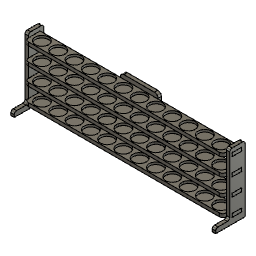
BDPRackv2 (Autodesk Fusion 360 design; units mm, degrees)
Autodesk Fusion 360 part; units mm, degrees
sketch "Sketch1" plane through (0, 0, 0) normal (0, 1, 0) x (1, 0, 0)
  line L0 (0, 0) -> (1066.8, 0)
  line L1 (1066.8, 0) -> (1066.8, -82.55)
  line L2 (1066.8, -82.55) -> (0, -82.55)
  line L3 (0, -82.55) -> (0, 0)
  line L4 (0, 0) -> (-18.288, 0)
  line L5 (-18.288, 0) -> (-18.288, -50.8)
  line L6 (-18.288, -50.8) -> (0, -50.8)
  line L7 (0, -50.8) -> (0, 0)
  line L8 (1066.8, 0) -> (1085.088, 0)
  line L9 (1085.088, 0) -> (1085.088, -50.8)
  line L10 (1085.088, -50.8) -> (1066.8, -50.8)
  line L11 (1066.8, -50.8) -> (1066.8, 0)
  line L12 (0, 0) -> (50.8, 0) construction
  line L13 (50.8, 0) -> (50.8, -41.275) construction
  circle A0 centre (50.8, -41.275) radius 36.195
  circle A1 centre (138.5455, -41.275) radius 36.195
  circle A2 centre (226.2909, -41.275) radius 36.195
  circle A3 centre (314.0364, -41.275) radius 36.195
  circle A4 centre (401.7818, -41.275) radius 36.195
  circle A5 centre (489.5273, -41.275) radius 36.195
  circle A6 centre (577.2727, -41.275) radius 36.195
  circle A7 centre (665.0182, -41.275) radius 36.195
  circle A8 centre (752.7636, -41.275) radius 36.195
  circle A9 centre (840.5091, -41.275) radius 36.195
  circle A10 centre (928.2545, -41.275) radius 36.195
  circle A11 centre (1016, -41.275) radius 36.195
  dimension "d1" = 1066.8
  dimension "d2" = 82.55
  dimension "d3" = 18.288
  dimension "d4" = 50.8
  dimension "d5" = 18.288
  dimension "d6" = 50.8
  dimension "d7" = 50.8
  dimension "d8" = 41.275
  dimension "d10" = 72.39
  dimension "d13" = 965.2
  dimension "d14" = 0
  constraint horizontal L0
  constraint vertical L1
  constraint horizontal L2
  constraint vertical L3
  constraint coincident L0.start L3.end
  constraint horizontal L4
  constraint vertical L5
  constraint horizontal L6
  constraint vertical L7
  constraint horizontal L8
  constraint vertical L9
  constraint horizontal L10
  constraint vertical L11
  constraint perpendicular L7 L12
  constraint perpendicular L0 L13
  constraint coincident L13.end A0.centre
  measures "d1" distance of L0.start L0.end
  measures "d2" distance of L0.start L2.end
  measures "d3" distance of L0.start L4.end
  measures "d4" distance of L0.start L6.end
  measures "d5" distance of L0.end L8.end
  measures "d6" distance of L0.end L10.end
  measures "d7" distance of L0.start L12.end
  measures "d8" distance of L12.end L13.end
  measures "d10" diameter of A0
extrude "Extrude1" add sketch "Sketch1" along normal blind 11.938 makes body 1 in component "Shelf"
sketch "Sketch2" plane through (0, 0, 0) normal (0, -1, 0) x (1, 0, 0)
  circle A0 centre (489.5273, 41.275) radius 36.195
  circle A1 centre (665.0182, 41.275) radius 36.195
  circle A2 centre (50.8, 41.275) radius 36.195
  circle A3 centre (928.2545, 41.275) radius 36.195
  circle A4 centre (226.2909, 41.275) radius 36.195
  circle A5 centre (314.0364, 41.275) radius 36.195
  circle A6 centre (401.7818, 41.275) radius 36.195
  circle A7 centre (138.5455, 41.275) radius 36.195
  circle A8 centre (752.7636, 41.275) radius 36.195
  circle A9 centre (1016, 41.275) radius 36.195
  circle A10 centre (840.5091, 41.275) radius 36.195
  circle A11 centre (577.2727, 41.275) radius 36.195
  line L0 (-18.288, 0) -> (1085.088, 0)
  line L1 (1085.088, 0) -> (1085.088, 50.8)
  line L2 (1085.088, 50.8) -> (1066.8, 50.8)
  line L3 (1066.8, 50.8) -> (1066.8, 82.55)
  line L4 (1066.8, 82.55) -> (0, 82.55)
  line L5 (0, 82.55) -> (0, 50.8)
  line L6 (0, 50.8) -> (-18.288, 50.8)
  line L7 (-18.288, 50.8) -> (-18.288, 0)
extrude "Extrude2" add sketch "Sketch2" along normal blind 6.35 contours A0 | A1 | A2 | A3 | A4 | A5 | A6 | A7 | A8 | A9 | A10 | A11 | L0 L1 L2 L3 L4 L5 L6 L7 bodies 1 in component "Shelf"
ref_plane "WorkPlane1" through (0, -6.35, 50.8) normal (0, 1, 0) x (-1, 0, 0)
sketch "Sketch3" plane through (0, -6.35, 50.8) normal (0, 1, 0) x (-1, 0, 0)
  line L0 (18.288, 0) -> (0, 0) construction
  line L1 (0, 0) -> (0, 31.75) construction
  line L2 (0, 0) -> (2.2451, 2.2451) construction
  circle A0 centre (2.2451, 2.2451) radius 3.175
  dimension "d20" = 3.175
  constraint coincident L0.end L1.start
  constraint coincident L0.end A0
  measures "d20" distance of L0.end L2.end
sweep "Sweep1" cut kept parallel profiles "Sketch3" along 1 edges at (0, 2.794, 50.8) section 1 on bodies 1 bodies 1 in component "Shelf"
ref_plane "WorkPlane2" through (1066.8, -6.35, 50.8) normal (0, 1, 0) x (-1, 0, 0)
sketch "Sketch4" plane through (1066.8, -6.35, 50.8) normal (0, 1, 0) x (-1, 0, 0)
  line L0 (0, 31.75) -> (0, 0) construction
  line L1 (0, 0) -> (-18.288, 0) construction
  line L2 (0, 0) -> (-2.2451, 2.2451) construction
  circle A0 centre (-2.2451, 2.2451) radius 3.175
  dimension "d28" = 3.175
  constraint coincident L0.end L1.start
  constraint coincident L0.end A0
  measures "d28" distance of L0.end L2.end
sweep "Sweep2" cut kept parallel profiles "Sketch4" along 1 edges at (1066.8, 2.794, 50.8) section 1 on bodies 1 bodies 1 in component "Shelf"
fillet "Fillet1" radius 19.05 2 edges at (1066.8, 2.794, 82.55) (0, 2.794, 82.55) on bodies 1 in component "Shelf"
sketch "Sketch5" plane through (1066.8, 0, 0) normal (1, 0, 0) x (0, 0, -1)
  line L0 (-63.5, 11.938) -> (-63.5, -6.35)
  line L1 (-63.5, -6.35) -> (-63.5, -12.7)
  line L2 (-63.5, -12.7) -> (-139.7, -12.7)
  line L3 (-139.7, -12.7) -> (-139.7, -38.1)
  line L4 (-139.7, -38.1) -> (19.05, -38.1)
  line L5 (19.05, -38.1) -> (19.05, 317.5)
  line L6 (19.05, -38.1) -> (19.05, 88.138) construction
  line L7 (19.05, 88.138) -> (19.05, 182.626) construction
  line L8 (19.05, 182.626) -> (19.05, 277.114) construction
  line L9 (19.05, 277.114) -> (0, 277.114) construction
  line L10 (19.05, 182.626) -> (0, 182.626) construction
  line L11 (19.05, 88.138) -> (0, 88.138) construction
  line L12 (0, 277.114) -> (-50.8, 277.114)
  line L13 (-50.8, 277.114) -> (-50.8, 295.402)
  line L14 (-50.8, 295.402) -> (0, 295.402)
  line L15 (0, 295.402) -> (0, 277.114)
  line L16 (0, 182.626) -> (-50.8, 182.626)
  line L17 (-50.8, 182.626) -> (-50.8, 200.914)
  line L18 (-50.8, 200.914) -> (0, 200.914)
  line L19 (0, 200.914) -> (0, 182.626)
  line L20 (0, 88.138) -> (-50.8, 88.138)
  line L21 (-50.8, 88.138) -> (-50.8, 106.426)
  line L22 (-50.8, 106.426) -> (0, 106.426)
  line L23 (0, 106.426) -> (0, 88.138)
  line L24 (19.05, -38.1) -> (19.05, -6.35) construction
  line L25 (19.05, -6.35) -> (19.05, -7.0008) construction
  line L26 (19.05, -6.35) -> (0, -6.35) construction
  line L27 (0, -6.35) -> (-50.8, -6.35)
  line L28 (-50.8, -6.35) -> (-50.8, 11.938)
  line L29 (-50.8, 11.938) -> (0, 11.938)
  line L30 (0, 11.938) -> (0, -6.35)
  line L31 (-63.5, -38.1) -> (-63.5, 317.5) construction
  line L32 (-63.5, 11.938) -> (-63.5, 317.5)
  line L33 (-63.5, 317.5) -> (19.05, 317.5)
  dimension "d37" = 6.35
  dimension "d38" = 76.2
  dimension "d39" = 25.4
  dimension "d40" = 158.75
  dimension "d41" = 355.6
  dimension "d42" = 126.238
  dimension "d43" = 94.488
  dimension "d44" = 94.488
  dimension "d45" = 19.05
  dimension "d46" = 19.05
  dimension "d47" = 19.05
  dimension "d48" = 50.8
  dimension "d49" = 18.288
  dimension "d50" = 50.8
  dimension "d51" = 18.288
  dimension "d52" = 50.8
  dimension "d53" = 18.288
  dimension "d54" = 31.75
  dimension "d55" = 19.05
  dimension "d56" = 18.288
  dimension "d57" = 355.6
  constraint coincident L0.end L1.start
  constraint parallel L0 L1
  constraint perpendicular L1 L2
  constraint perpendicular L2 L3
  constraint perpendicular L3 L4
  constraint perpendicular L4 L5
  constraint perpendicular L4 L6
  constraint parallel L5 L7
  constraint parallel L5 L8
  constraint perpendicular L8 L9
  constraint perpendicular L8 L10
  constraint perpendicular L6 L11
  constraint horizontal L12
  constraint vertical L13
  constraint horizontal L14
  constraint vertical L15
  constraint horizontal L16
  constraint vertical L17
  constraint horizontal L18
  constraint vertical L19
  constraint horizontal L20
  constraint vertical L21
  constraint horizontal L22
  constraint vertical L23
  constraint perpendicular L4 L24
  constraint coincident L6 L25.end
  constraint perpendicular L24 L26
  constraint horizontal L27
  constraint vertical L28
  constraint horizontal L29
  constraint vertical L30
  constraint coincident L4 L31.start
  constraint perpendicular L4 L31
  constraint coincident L0.start L32.start
  constraint perpendicular L20 L32
  constraint perpendicular L5 L33
  measures "d37" distance of L0.end L1.end
  measures "d38" distance of L1.end L2.end
  measures "d39" distance of L2.end L3.end
  measures "d40" distance of L3.end L4.end
  measures "d41" distance of L4.end L5.end
  measures "d42" distance of L4.end L6.end
  measures "d43" distance of L6.end L7.end
  measures "d44" distance of L7.end L8.end
  measures "d45" distance of L8.end L9.end
  measures "d46" distance of L7.end L10.end
  measures "d47" distance of L6.end L11.end
  measures "d48" distance of L9.end L12.end
  measures "d49" distance of L9.end L14.end
  measures "d50" distance of L10.end L16.end
  measures "d51" distance of L10.end L18.end
  measures "d52" distance of L11.end L20.end
  measures "d53" distance of L11.end L22.end
  measures "d54" distance of L4.end L24.end
  measures "d55" distance of L24.end L26.end
  measures "d56" distance of L26.end L29.end
  measures "d57" distance of L31.start L31.end
extrude "Extrude1'" add sketch "Sketch5" along normal blind 18.288 separate body makes body 2 in component "Side"
fillet "Fillet1'" radius 12.7 4 edges at (1075.944, -12.7, 63.5) (1075.944, -12.7, 139.7) (1075.944, 317.5, 63.5) (1075.944, 317.5, -19.05) on bodies 2 in component "Side"
sketch "Sketch6" plane through (0, 0, 0) normal (0, 0, -1) x (-1, 0, 0)
  line L0 (18.288, -6.35) -> (18.288, 11.938)
  line L1 (18.288, 11.938) -> (-1085.088, 11.938)
  line L2 (-1085.088, 11.938) -> (-1085.088, -6.35)
  line L3 (-1085.088, -6.35) -> (18.288, -6.35)
  line L4 (-533.4, 11.938) -> (-533.4, 2.794) construction
  line L5 (-457.2, -6.35) -> (-609.6, -6.35)
  line L6 (-609.6, -6.35) -> (-609.6, 11.938)
  line L7 (-609.6, 11.938) -> (-457.2, 11.938)
  line L8 (-457.2, 11.938) -> (-457.2, -6.35)
  line L9 (-457.2, -6.35) -> (-609.6, 11.938) construction
  line L10 (-609.6, -6.35) -> (-457.2, 11.938) construction
  point P0 (-533.4, 2.794)
  dimension "d62" = 9.144
  dimension "d63" = 152.4
  constraint midpoint L1 L4.start
  constraint perpendicular L1 L4
  constraint horizontal L5
  constraint perpendicular L5 L6
  constraint parallel L5 L7
  constraint parallel L6 L8
  constraint coincident L9 P0
  constraint coincident L10 P0
  constraint coincident P0 L4.end
  measures "d62" distance of L4.start P0
  measures "d63" distance of L6.end L7.end
extrude "Extrude3" add sketch "Sketch6" along normal blind 18.288 contours L1 L3 L5 L6 L7 L8 bodies 1 in component "Shelf"
ref_plane "WorkPlane3" through (1066.8, 295.402, 0) normal (1, 0, 0) x (0, 1, 0)
sketch "Sketch7" plane through (1066.8, 295.402, 0) normal (1, 0, 0) x (0, 1, 0)
  line L0 (0, 50.8) -> (0, 0) construction
  line L1 (0, 0) -> (-18.288, 0) construction
  line L2 (0, 0) -> (-2.2451, 2.2451) construction
  circle A0 centre (-2.2451, 2.2451) radius 3.175
  dimension "d67" = 3.175
  constraint coincident L0.end L1.start
  constraint coincident L0.end A0
  measures "d67" distance of L0.end L2.end
sweep "Sweep1'" cut kept parallel profiles "Sketch7" along 1 edges at (1075.944, 295.402, 0) section 1 on bodies 2 bodies 2 in component "Side"
ref_plane "WorkPlane4" through (1066.8, 200.914, 0) normal (1, 0, 0) x (0, 1, 0)
sketch "Sketch8" plane through (1066.8, 200.914, 0) normal (1, 0, 0) x (0, 1, 0)
  line L0 (0, 50.8) -> (0, 0) construction
  line L1 (0, 0) -> (-18.288, 0) construction
  line L2 (0, 0) -> (-2.2451, 2.2451) construction
  circle A0 centre (-2.2451, 2.2451) radius 3.175
  dimension "d75" = 3.175
  constraint coincident L0.end L1.start
  constraint coincident L0.end A0
  measures "d75" distance of L0.end L2.end
sweep "Sweep2'" cut kept parallel profiles "Sketch8" along 1 edges at (1075.944, 200.914, 0) section 1 on bodies 2 bodies 2 in component "Side"
ref_plane "WorkPlane5" through (1066.8, 11.938, 0) normal (1, 0, 0) x (0, 1, 0)
sketch "Sketch9" plane through (1066.8, 11.938, 0) normal (1, 0, 0) x (0, 1, 0)
  line L0 (0, 50.8) -> (0, 0) construction
  line L1 (0, 0) -> (-18.288, 0) construction
  line L2 (0, 0) -> (-2.2451, 2.2451) construction
  circle A0 centre (-2.2451, 2.2451) radius 3.175
  dimension "d83" = 3.175
  constraint coincident L0.end L1.start
  constraint coincident L0.end A0
  measures "d83" distance of L0.end L2.end
sweep "Sweep3" cut kept parallel profiles "Sketch9" along 1 edges at (1075.944, 11.938, 0) section 1 on bodies 2 bodies 2 in component "Side"
ref_plane "WorkPlane6" through (1066.8, 106.426, 0) normal (1, 0, 0) x (0, 1, 0)
sketch "Sketch10" plane through (1066.8, 106.426, 0) normal (1, 0, 0) x (0, 1, 0)
  line L0 (0, 50.8) -> (0, 0) construction
  line L1 (0, 0) -> (-18.288, 0) construction
  line L2 (0, 0) -> (-2.2451, 2.2451) construction
  circle A0 centre (-2.2451, 2.2451) radius 3.175
  dimension "d91" = 3.175
  constraint coincident L0.end L1.start
  constraint coincident L0.end A0
  measures "d91" distance of L0.end L2.end
sweep "Sweep4" cut kept parallel profiles "Sketch10" along 1 edges at (1075.944, 106.426, 0) section 1 on bodies 2 bodies 2 in component "Side"
ref_plane "WorkPlane7" through (1066.8, 11.938, 50.8) normal (1, 0, 0) x (0, 1, 0)
sketch "Sketch11" plane through (1066.8, 11.938, 50.8) normal (1, 0, 0) x (0, 1, 0)
  line L0 (0, 0) -> (0, -46.3099) construction
  line L1 (-18.288, 0) -> (0, 0) construction
  line L2 (0, 0) -> (-2.2451, -2.2451) construction
  circle A0 centre (-2.2451, -2.2451) radius 3.175
  dimension "d99" = 3.175
  constraint coincident L0.start L1.end
  constraint coincident L0.start A0
  measures "d99" distance of L0.start L2.end
sweep "Sweep5" cut kept parallel profiles "Sketch11" along 1 edges at (1075.944, 11.938, 50.8) section 1 on bodies 2 bodies 2 in component "Side"
ref_plane "WorkPlane8" through (1066.8, 106.426, 50.8) normal (1, 0, 0) x (0, 1, 0)
sketch "Sketch12" plane through (1066.8, 106.426, 50.8) normal (1, 0, 0) x (0, 1, 0)
  line L0 (0, 0) -> (0, -46.3099) construction
  line L1 (-18.288, 0) -> (0, 0) construction
  line L2 (0, 0) -> (-2.2451, -2.2451) construction
  circle A0 centre (-2.2451, -2.2451) radius 3.175
  dimension "d107" = 3.175
  constraint coincident L0.start L1.end
  constraint coincident L0.start A0
  measures "d107" distance of L0.start L2.end
sweep "Sweep6" cut kept parallel profiles "Sketch12" along 1 edges at (1075.944, 106.426, 50.8) section 1 on bodies 2 bodies 2 in component "Side"
ref_plane "WorkPlane9" through (1066.8, 295.402, 50.8) normal (1, 0, 0) x (0, 1, 0)
sketch "Sketch13" plane through (1066.8, 295.402, 50.8) normal (1, 0, 0) x (0, 1, 0)
  line L0 (0, 0) -> (0, -46.3099) construction
  line L1 (-18.288, 0) -> (0, 0) construction
  line L2 (0, 0) -> (-2.2451, -2.2451) construction
  circle A0 centre (-2.2451, -2.2451) radius 3.175
  dimension "d115" = 3.175
  constraint coincident L0.start L1.end
  constraint coincident L0.start A0
  measures "d115" distance of L0.start L2.end
sweep "Sweep7" cut kept parallel profiles "Sketch13" along 1 edges at (1075.944, 295.402, 50.8) section 1 on bodies 2 bodies 2 in component "Side"
ref_plane "WorkPlane10" through (1066.8, 200.914, 50.8) normal (1, 0, 0) x (0, 1, 0)
sketch "Sketch14" plane through (1066.8, 200.914, 50.8) normal (1, 0, 0) x (0, 1, 0)
  line L0 (0, 0) -> (0, -46.3099) construction
  line L1 (-18.288, 0) -> (0, 0) construction
  line L2 (0, 0) -> (-2.2451, -2.2451) construction
  circle A0 centre (-2.2451, -2.2451) radius 3.175
  dimension "d123" = 3.175
  constraint coincident L0.start L1.end
  constraint coincident L0.start A0
  measures "d123" distance of L0.start L2.end
sweep "Sweep8" cut kept parallel profiles "Sketch14" along 1 edges at (1075.944, 200.914, 50.8) section 1 on bodies 2 bodies 2 in component "Side"
ref_plane "WorkPlane11" through (1066.8, 277.114, 0) normal (1, 0, 0) x (0, 1, 0)
sketch "Sketch15" plane through (1066.8, 277.114, 0) normal (1, 0, 0) x (0, 1, 0)
  line L0 (13.7979, 0) -> (0, 0) construction
  line L1 (0, 0) -> (0, 50.8) construction
  line L2 (0, 0) -> (2.2451, 2.2451) construction
  circle A0 centre (2.2451, 2.2451) radius 3.175
  dimension "d131" = 3.175
  constraint coincident L0.end L1.start
  constraint coincident L0.end A0
  measures "d131" distance of L0.end L2.end
sweep "Sweep9" cut kept parallel profiles "Sketch15" along 1 edges at (1075.944, 277.114, 0) section 1 on bodies 2 bodies 2 in component "Side"
ref_plane "WorkPlane12" through (1066.8, 182.626, 0) normal (1, 0, 0) x (0, 1, 0)
sketch "Sketch16" plane through (1066.8, 182.626, 0) normal (1, 0, 0) x (0, 1, 0)
  line L0 (13.7979, 0) -> (0, 0) construction
  line L1 (0, 0) -> (0, 50.8) construction
  line L2 (0, 0) -> (2.2451, 2.2451) construction
  circle A0 centre (2.2451, 2.2451) radius 3.175
  dimension "d139" = 3.175
  constraint coincident L0.end L1.start
  constraint coincident L0.end A0
  measures "d139" distance of L0.end L2.end
sweep "Sweep10" cut kept parallel profiles "Sketch16" along 1 edges at (1075.944, 182.626, 0) section 1 on bodies 2 bodies 2 in component "Side"
ref_plane "WorkPlane13" through (1066.8, 88.138, 0) normal (1, 0, 0) x (0, 1, 0)
sketch "Sketch17" plane through (1066.8, 88.138, 0) normal (1, 0, 0) x (0, 1, 0)
  line L0 (13.7979, 0) -> (0, 0) construction
  line L1 (0, 0) -> (0, 50.8) construction
  line L2 (0, 0) -> (2.2451, 2.2451) construction
  circle A0 centre (2.2451, 2.2451) radius 3.175
  dimension "d147" = 3.175
  constraint coincident L0.end L1.start
  constraint coincident L0.end A0
  measures "d147" distance of L0.end L2.end
sweep "Sweep11" cut kept parallel profiles "Sketch17" along 1 edges at (1075.944, 88.138, 0) section 1 on bodies 2 bodies 2 in component "Side"
ref_plane "WorkPlane14" through (1066.8, -6.35, 0) normal (1, 0, 0) x (0, 1, 0)
sketch "Sketch18" plane through (1066.8, -6.35, 0) normal (1, 0, 0) x (0, 1, 0)
  line L0 (13.7979, 0) -> (0, 0) construction
  line L1 (0, 0) -> (0, 50.8) construction
  line L2 (0, 0) -> (2.2451, 2.2451) construction
  circle A0 centre (2.2451, 2.2451) radius 3.175
  dimension "d155" = 3.175
  constraint coincident L0.end L1.start
  constraint coincident L0.end A0
  measures "d155" distance of L0.end L2.end
sweep "Sweep12" cut kept parallel profiles "Sketch18" along 1 edges at (1075.944, -6.35, 0) section 1 on bodies 2 bodies 2 in component "Side"
ref_plane "WorkPlane15" through (1066.8, -6.35, 50.8) normal (1, 0, 0) x (0, 1, 0)
sketch "Sketch19" plane through (1066.8, -6.35, 50.8) normal (1, 0, 0) x (0, 1, 0)
  line L0 (0, -46.3099) -> (0, 0) construction
  line L1 (0, 0) -> (13.7979, 0) construction
  line L2 (0, 0) -> (2.2451, -2.2451) construction
  circle A0 centre (2.2451, -2.2451) radius 3.175
  dimension "d163" = 3.175
  constraint coincident L0.end L1.start
  constraint coincident L0.end A0
  measures "d163" distance of L0.end L2.end
sweep "Sweep13" cut kept parallel profiles "Sketch19" along 1 edges at (1075.944, -6.35, 50.8) section 1 on bodies 2 bodies 2 in component "Side"
ref_plane "WorkPlane16" through (1066.8, 88.138, 50.8) normal (1, 0, 0) x (0, 1, 0)
sketch "Sketch20" plane through (1066.8, 88.138, 50.8) normal (1, 0, 0) x (0, 1, 0)
  line L0 (0, -46.3099) -> (0, 0) construction
  line L1 (0, 0) -> (13.7979, 0) construction
  line L2 (0, 0) -> (2.2451, -2.2451) construction
  circle A0 centre (2.2451, -2.2451) radius 3.175
  dimension "d171" = 3.175
  constraint coincident L0.end L1.start
  constraint coincident L0.end A0
  measures "d171" distance of L0.end L2.end
sweep "Sweep14" cut kept parallel profiles "Sketch20" along 1 edges at (1075.944, 88.138, 50.8) section 1 on bodies 2 bodies 2 in component "Side"
ref_plane "WorkPlane17" through (1066.8, 182.626, 50.8) normal (1, 0, 0) x (0, 1, 0)
sketch "Sketch21" plane through (1066.8, 182.626, 50.8) normal (1, 0, 0) x (0, 1, 0)
  line L0 (0, -46.3099) -> (0, 0) construction
  line L1 (0, 0) -> (13.7979, 0) construction
  line L2 (0, 0) -> (2.2451, -2.2451) construction
  circle A0 centre (2.2451, -2.2451) radius 3.175
  dimension "d179" = 3.175
  constraint coincident L0.end L1.start
  constraint coincident L0.end A0
  measures "d179" distance of L0.end L2.end
sweep "Sweep15" cut kept parallel profiles "Sketch21" along 1 edges at (1075.944, 182.626, 50.8) section 1 on bodies 2 bodies 2 in component "Side"
ref_plane "WorkPlane18" through (1066.8, 277.114, 50.8) normal (1, 0, 0) x (0, 1, 0)
sketch "Sketch22" plane through (1066.8, 277.114, 50.8) normal (1, 0, 0) x (0, 1, 0)
  line L0 (0, -46.3099) -> (0, 0) construction
  line L1 (0, 0) -> (13.7979, 0) construction
  line L2 (0, 0) -> (2.2451, -2.2451) construction
  circle A0 centre (2.2451, -2.2451) radius 3.175
  dimension "d187" = 3.175
  constraint coincident L0.end L1.start
  constraint coincident L0.end A0
  measures "d187" distance of L0.end L2.end
sweep "Sweep16" cut kept parallel profiles "Sketch22" along 1 edges at (1075.944, 277.114, 50.8) section 1 on bodies 2 bodies 2 in component "Side"
ref_plane "WorkPlane19" through (457.2, 11.938, 0) normal (0, -1, 0) x (1, 0, 0)
sketch "Sketch23" plane through (457.2, 11.938, 0) normal (0, -1, 0) x (1, 0, 0)
  line L0 (-475.488, 0) -> (0, 0) construction
  line L1 (0, 0) -> (0, -18.288) construction
  line L2 (0, 0) -> (-2.2451, -2.2451) construction
  circle A0 centre (-2.2451, -2.2451) radius 3.175
  dimension "d195" = 3.175
  constraint coincident L0.end L1.start
  constraint coincident L0.end A0
  measures "d195" distance of L0.end L2.end
sweep "Sweep3'" cut kept parallel profiles "Sketch23" along 1 edges at (457.2, 2.794, 0) section 1 on bodies 1 bodies 1 in component "Shelf"
ref_plane "WorkPlane20" through (609.6, -6.35, 0) normal (0, 1, 0) x (-1, 0, 0)
sketch "Sketch24" plane through (609.6, -6.35, 0) normal (0, 1, 0) x (-1, 0, 0)
  line L0 (-475.488, 0) -> (0, 0) construction
  line L1 (0, 0) -> (0, -18.288) construction
  line L2 (0, 0) -> (-2.2451, -2.2451) construction
  circle A0 centre (-2.2451, -2.2451) radius 3.175
  dimension "d203" = 3.175
  constraint coincident L0.end L1.start
  constraint coincident L0.end A0
  measures "d203" distance of L0.end L2.end
sweep "Sweep4'" cut kept parallel profiles "Sketch24" along 1 edges at (609.6, 2.794, 0) section 1 on bodies 1 bodies 1 in component "Shelf"
sketch "Sketch25" plane through (0, 0, -18.288) normal (0, 0, -1) x (-1, 0, 0)
  line L0 (-457.2, 11.938) -> (-609.6, 11.938)
  line L1 (-609.6, 11.938) -> (-609.6, -6.35)
  line L2 (-609.6, -6.35) -> (-457.2, -6.35)
  line L3 (-457.2, -6.35) -> (-457.2, 11.938)
  line L4 (-533.4, 11.938) -> (-533.4, 2.794) construction
  line L5 (-533.4, 2.794) -> (-533.4, 97.282) construction
  line L6 (-533.4, 97.282) -> (-533.4, 191.77) construction
  line L7 (-533.4, 191.77) -> (-533.4, 286.258) construction
  line L8 (-533.4, 2.794) -> (-533.4, -6.35) construction
  line L9 (-533.4, -6.35) -> (-533.4, -38.1) construction
  line L10 (-533.4, -38.1) -> (-635, -38.1) construction
  line L11 (-635, -38.1) -> (-431.8, -38.1)
  line L12 (-431.8, -38.1) -> (-431.8, 317.5)
  line L13 (-431.8, 317.5) -> (-635, 317.5)
  line L14 (-635, 317.5) -> (-635, -38.1)
  line L15 (-457.2, 277.114) -> (-609.6, 277.114)
  line L16 (-609.6, 277.114) -> (-609.6, 295.402)
  line L17 (-609.6, 295.402) -> (-457.2, 295.402)
  line L18 (-457.2, 295.402) -> (-457.2, 277.114)
  line L19 (-457.2, 277.114) -> (-609.6, 295.402) construction
  line L20 (-609.6, 277.114) -> (-457.2, 295.402) construction
  line L21 (-457.2, 182.626) -> (-609.6, 182.626)
  line L22 (-609.6, 182.626) -> (-609.6, 200.914)
  line L23 (-609.6, 200.914) -> (-457.2, 200.914)
  line L24 (-457.2, 200.914) -> (-457.2, 182.626)
  line L25 (-457.2, 182.626) -> (-609.6, 200.914) construction
  line L26 (-609.6, 182.626) -> (-457.2, 200.914) construction
  line L27 (-457.2, 88.138) -> (-609.6, 88.138)
  line L28 (-609.6, 88.138) -> (-609.6, 106.426)
  line L29 (-609.6, 106.426) -> (-457.2, 106.426)
  line L30 (-457.2, 106.426) -> (-457.2, 88.138)
  line L31 (-457.2, 88.138) -> (-609.6, 106.426) construction
  line L32 (-609.6, 88.138) -> (-457.2, 106.426) construction
  line L33 (-457.2, -6.35) -> (-609.6, -6.35)
  line L34 (-609.6, -6.35) -> (-609.6, 11.938)
  line L35 (-609.6, 11.938) -> (-457.2, 11.938)
  line L36 (-457.2, 11.938) -> (-457.2, -6.35)
  line L37 (-457.2, -6.35) -> (-609.6, 11.938) construction
  line L38 (-609.6, -6.35) -> (-457.2, 11.938) construction
  point P0 (-533.4, 286.258)
  point P1 (-533.4, 191.77)
  point P2 (-533.4, 97.282)
  point P3 (-533.4, 2.794)
  dimension "d210" = 9.144
  dimension "d211" = 94.488
  dimension "d212" = 94.488
  dimension "d213" = 94.488
  dimension "d214" = 31.75
  dimension "d215" = 101.6
  dimension "d216" = 203.2
  dimension "d217" = 355.6
  dimension "d218" = 152.4
  dimension "d219" = 18.288
  dimension "d220" = 152.4
  dimension "d221" = 18.288
  dimension "d222" = 152.4
  dimension "d223" = 18.288
  dimension "d224" = 152.4
  constraint midpoint L0 L4.start
  constraint perpendicular L0 L4
  constraint perpendicular L0 L5
  constraint vertical L6
  constraint parallel L6 L7
  constraint midpoint L2 L8.end
  constraint perpendicular L2 L9
  constraint perpendicular L9 L10
  constraint horizontal L11
  constraint vertical L12
  constraint horizontal L13
  constraint vertical L14
  constraint horizontal L15
  constraint perpendicular L15 L16
  constraint parallel L15 L17
  constraint parallel L16 L18
  constraint coincident L19 P0
  constraint coincident L20 P0
  constraint coincident P0 L7.end
  constraint horizontal L21
  constraint perpendicular L21 L22
  constraint parallel L21 L23
  constraint parallel L22 L24
  constraint coincident L25 P1
  constraint coincident L26 P1
  constraint coincident P1 L6.end
  constraint horizontal L27
  constraint perpendicular L27 L28
  constraint parallel L27 L29
  constraint parallel L28 L30
  constraint coincident L31 P2
  constraint coincident L32 P2
  constraint coincident P2 L5.end
  constraint horizontal L33
  constraint perpendicular L33 L34
  constraint parallel L33 L35
  constraint parallel L34 L36
  constraint coincident L37 P3
  constraint coincident L38 P3
  constraint coincident P3 L4.end
  measures "d210" distance of L4.start P3
  measures "d211" distance of P3 P2
  measures "d212" distance of P2 P1
  measures "d213" distance of P1 P0
  measures "d214" distance of L8.end L9.end
  measures "d215" distance of L9.end L10.end
  measures "d216" distance of L10.end L11.end
  measures "d217" distance of L10.end L13.end
  measures "d218" distance of L16.end L17.end
  measures "d219" distance of L15.end L16.end
  measures "d220" distance of L22.end L23.end
  measures "d221" distance of L21.end L22.end
  measures "d222" distance of L28.end L29.end
  measures "d223" distance of L27.end L28.end
  measures "d224" distance of L0.end L0.start
extrude "Extrude1''" add sketch "Sketch25" against normal blind 18.288 separate body makes body 3 in component "Back"
fillet "Fillet1''" radius 19.05 2 edges at (635, 317.5, -9.144) (431.8, 317.5, -9.144) on bodies 3 in component "Back"
ref_plane "WorkPlane21" through (457.2, 277.114, -18.288) normal (0, 0, 1) x (1, 0, 0)
sketch "Sketch26" plane through (457.2, 277.114, -18.288) normal (0, 0, 1) x (1, 0, 0)
  line L0 (0, 0) -> (152.4, 0) construction
  line L1 (0, 18.288) -> (0, 0) construction
  line L2 (0, 0) -> (2.2451, 2.2451) construction
  circle A0 centre (2.2451, 2.2451) radius 3.175
  dimension "d230" = 3.175
  constraint coincident L0.start L1.end
  constraint coincident L0.start A0
  measures "d230" distance of L0.start L2.end
sweep "Sweep1''" cut kept parallel profiles "Sketch26" along 1 edges at (457.2, 277.114, -9.144) section 1 on bodies 3 bodies 3 in component "Back"
ref_plane "WorkPlane22" through (457.2, 182.626, -18.288) normal (0, 0, 1) x (1, 0, 0)
sketch "Sketch27" plane through (457.2, 182.626, -18.288) normal (0, 0, 1) x (1, 0, 0)
  line L0 (0, 0) -> (152.4, 0) construction
  line L1 (0, 18.288) -> (0, 0) construction
  line L2 (0, 0) -> (2.2451, 2.2451) construction
  circle A0 centre (2.2451, 2.2451) radius 3.175
  dimension "d238" = 3.175
  constraint coincident L0.start L1.end
  constraint coincident L0.start A0
  measures "d238" distance of L0.start L2.end
sweep "Sweep2''" cut kept parallel profiles "Sketch27" along 1 edges at (457.2, 182.626, -9.144) section 1 on bodies 3 bodies 3 in component "Back"
ref_plane "WorkPlane23" through (457.2, 88.138, -18.288) normal (0, 0, 1) x (1, 0, 0)
sketch "Sketch28" plane through (457.2, 88.138, -18.288) normal (0, 0, 1) x (1, 0, 0)
  line L0 (0, 0) -> (152.4, 0) construction
  line L1 (0, 18.288) -> (0, 0) construction
  line L2 (0, 0) -> (2.2451, 2.2451) construction
  circle A0 centre (2.2451, 2.2451) radius 3.175
  dimension "d246" = 3.175
  constraint coincident L0.start L1.end
  constraint coincident L0.start A0
  measures "d246" distance of L0.start L2.end
sweep "Sweep3''" cut kept parallel profiles "Sketch28" along 1 edges at (457.2, 88.138, -9.144) section 1 on bodies 3 bodies 3 in component "Back"
ref_plane "WorkPlane24" through (457.2, -6.35, -18.288) normal (0, 0, 1) x (1, 0, 0)
sketch "Sketch29" plane through (457.2, -6.35, -18.288) normal (0, 0, 1) x (1, 0, 0)
  line L0 (0, 0) -> (152.4, 0) construction
  line L1 (0, 18.288) -> (0, 0) construction
  line L2 (0, 0) -> (2.2451, 2.2451) construction
  circle A0 centre (2.2451, 2.2451) radius 3.175
  dimension "d254" = 3.175
  constraint coincident L0.start L1.end
  constraint coincident L0.start A0
  measures "d254" distance of L0.start L2.end
sweep "Sweep4''" cut kept parallel profiles "Sketch29" along 1 edges at (457.2, -6.35, -9.144) section 1 on bodies 3 bodies 3 in component "Back"
ref_plane "WorkPlane25" through (609.6, -6.35, -18.288) normal (0, 0, 1) x (1, 0, 0)
sketch "Sketch30" plane through (609.6, -6.35, -18.288) normal (0, 0, 1) x (1, 0, 0)
  line L0 (0, 0) -> (0, 18.288) construction
  line L1 (-147.9099, 0) -> (0, 0) construction
  line L2 (0, 0) -> (-2.2451, 2.2451) construction
  circle A0 centre (-2.2451, 2.2451) radius 3.175
  dimension "d262" = 3.175
  constraint coincident L0.start L1.end
  constraint coincident L0.start A0
  measures "d262" distance of L0.start L2.end
sweep "Sweep5'" cut kept parallel profiles "Sketch30" along 1 edges at (609.6, -6.35, -9.144) section 1 on bodies 3 bodies 3 in component "Back"
ref_plane "WorkPlane26" through (609.6, 88.138, -18.288) normal (0, 0, 1) x (1, 0, 0)
sketch "Sketch31" plane through (609.6, 88.138, -18.288) normal (0, 0, 1) x (1, 0, 0)
  line L0 (0, 0) -> (0, 18.288) construction
  line L1 (-147.9099, 0) -> (0, 0) construction
  line L2 (0, 0) -> (-2.2451, 2.2451) construction
  circle A0 centre (-2.2451, 2.2451) radius 3.175
  dimension "d270" = 3.175
  constraint coincident L0.start L1.end
  constraint coincident L0.start A0
  measures "d270" distance of L0.start L2.end
sweep "Sweep6'" cut kept parallel profiles "Sketch31" along 1 edges at (609.6, 88.138, -9.144) section 1 on bodies 3 bodies 3 in component "Back"
ref_plane "WorkPlane27" through (609.6, 182.626, -18.288) normal (0, 0, 1) x (1, 0, 0)
sketch "Sketch32" plane through (609.6, 182.626, -18.288) normal (0, 0, 1) x (1, 0, 0)
  line L0 (0, 0) -> (0, 18.288) construction
  line L1 (-147.9099, 0) -> (0, 0) construction
  line L2 (0, 0) -> (-2.2451, 2.2451) construction
  circle A0 centre (-2.2451, 2.2451) radius 3.175
  dimension "d278" = 3.175
  constraint coincident L0.start L1.end
  constraint coincident L0.start A0
  measures "d278" distance of L0.start L2.end
sweep "Sweep7'" cut kept parallel profiles "Sketch32" along 1 edges at (609.6, 182.626, -9.144) section 1 on bodies 3 bodies 3 in component "Back"
ref_plane "WorkPlane28" through (609.6, 277.114, -18.288) normal (0, 0, 1) x (1, 0, 0)
sketch "Sketch33" plane through (609.6, 277.114, -18.288) normal (0, 0, 1) x (1, 0, 0)
  line L0 (0, 0) -> (0, 18.288) construction
  line L1 (-147.9099, 0) -> (0, 0) construction
  line L2 (0, 0) -> (-2.2451, 2.2451) construction
  circle A0 centre (-2.2451, 2.2451) radius 3.175
  dimension "d286" = 3.175
  constraint coincident L0.start L1.end
  constraint coincident L0.start A0
  measures "d286" distance of L0.start L2.end
sweep "Sweep8'" cut kept parallel profiles "Sketch33" along 1 edges at (609.6, 277.114, -9.144) section 1 on bodies 3 bodies 3 in component "Back"
ref_plane "WorkPlane29" through (609.6, 295.402, -18.288) normal (0, 0, 1) x (1, 0, 0)
sketch "Sketch34" plane through (609.6, 295.402, -18.288) normal (0, 0, 1) x (1, 0, 0)
  line L0 (0, 0) -> (-152.4, 0) construction
  line L1 (0, -13.7979) -> (0, 0) construction
  line L2 (0, 0) -> (-2.2451, -2.2451) construction
  circle A0 centre (-2.2451, -2.2451) radius 3.175
  dimension "d294" = 3.175
  constraint coincident L0.start L1.end
  constraint coincident L0.start A0
  measures "d294" distance of L0.start L2.end
sweep "Sweep9'" cut kept parallel profiles "Sketch34" along 1 edges at (609.6, 295.402, -9.144) section 1 on bodies 3 bodies 3 in component "Back"
ref_plane "WorkPlane30" through (609.6, 200.914, -18.288) normal (0, 0, 1) x (1, 0, 0)
sketch "Sketch35" plane through (609.6, 200.914, -18.288) normal (0, 0, 1) x (1, 0, 0)
  line L0 (0, 0) -> (-152.4, 0) construction
  line L1 (0, -13.7979) -> (0, 0) construction
  line L2 (0, 0) -> (-2.2451, -2.2451) construction
  circle A0 centre (-2.2451, -2.2451) radius 3.175
  dimension "d302" = 3.175
  constraint coincident L0.start L1.end
  constraint coincident L0.start A0
  measures "d302" distance of L0.start L2.end
sweep "Sweep10'" cut kept parallel profiles "Sketch35" along 1 edges at (609.6, 200.914, -9.144) section 1 on bodies 3 bodies 3 in component "Back"
ref_plane "WorkPlane31" through (609.6, 106.426, -18.288) normal (0, 0, 1) x (1, 0, 0)
sketch "Sketch36" plane through (609.6, 106.426, -18.288) normal (0, 0, 1) x (1, 0, 0)
  line L0 (0, 0) -> (-152.4, 0) construction
  line L1 (0, -13.7979) -> (0, 0) construction
  line L2 (0, 0) -> (-2.2451, -2.2451) construction
  circle A0 centre (-2.2451, -2.2451) radius 3.175
  dimension "d310" = 3.175
  constraint coincident L0.start L1.end
  constraint coincident L0.start A0
  measures "d310" distance of L0.start L2.end
sweep "Sweep11'" cut kept parallel profiles "Sketch36" along 1 edges at (609.6, 106.426, -9.144) section 1 on bodies 3 bodies 3 in component "Back"
ref_plane "WorkPlane32" through (609.6, 11.938, -18.288) normal (0, 0, 1) x (1, 0, 0)
sketch "Sketch37" plane through (609.6, 11.938, -18.288) normal (0, 0, 1) x (1, 0, 0)
  line L0 (0, 0) -> (-152.4, 0) construction
  line L1 (0, -13.7979) -> (0, 0) construction
  line L2 (0, 0) -> (-2.2451, -2.2451) construction
  circle A0 centre (-2.2451, -2.2451) radius 3.175
  dimension "d318" = 3.175
  constraint coincident L0.start L1.end
  constraint coincident L0.start A0
  measures "d318" distance of L0.start L2.end
sweep "Sweep12'" cut kept parallel profiles "Sketch37" along 1 edges at (609.6, 11.938, -9.144) section 1 on bodies 3 bodies 3 in component "Back"
ref_plane "WorkPlane33" through (457.2, 295.402, -18.288) normal (0, 0, 1) x (1, 0, 0)
sketch "Sketch38" plane through (457.2, 295.402, -18.288) normal (0, 0, 1) x (1, 0, 0)
  line L0 (0, 0) -> (147.9099, 0) construction
  line L1 (0, -13.7979) -> (0, 0) construction
  line L2 (0, 0) -> (2.2451, -2.2451) construction
  circle A0 centre (2.2451, -2.2451) radius 3.175
  dimension "d326" = 3.175
  constraint coincident L0.start L1.end
  constraint coincident L0.start A0
  measures "d326" distance of L0.start L2.end
sweep "Sweep13'" cut kept parallel profiles "Sketch38" along 1 edges at (457.2, 295.402, -9.144) section 1 on bodies 3 bodies 3 in component "Back"
ref_plane "WorkPlane34" through (457.2, 200.914, -18.288) normal (0, 0, 1) x (1, 0, 0)
sketch "Sketch39" plane through (457.2, 200.914, -18.288) normal (0, 0, 1) x (1, 0, 0)
  line L0 (0, 0) -> (147.9099, 0) construction
  line L1 (0, -13.7979) -> (0, 0) construction
  line L2 (0, 0) -> (2.2451, -2.2451) construction
  circle A0 centre (2.2451, -2.2451) radius 3.175
  dimension "d334" = 3.175
  constraint coincident L0.start L1.end
  constraint coincident L0.start A0
  measures "d334" distance of L0.start L2.end
sweep "Sweep14'" cut kept parallel profiles "Sketch39" along 1 edges at (457.2, 200.914, -9.144) section 1 on bodies 3 bodies 3 in component "Back"
ref_plane "WorkPlane35" through (457.2, 106.426, -18.288) normal (0, 0, 1) x (1, 0, 0)
sketch "Sketch40" plane through (457.2, 106.426, -18.288) normal (0, 0, 1) x (1, 0, 0)
  line L0 (0, 0) -> (147.9099, 0) construction
  line L1 (0, -13.7979) -> (0, 0) construction
  line L2 (0, 0) -> (2.2451, -2.2451) construction
  circle A0 centre (2.2451, -2.2451) radius 3.175
  dimension "d342" = 3.175
  constraint coincident L0.start L1.end
  constraint coincident L0.start A0
  measures "d342" distance of L0.start L2.end
sweep "Sweep15'" cut kept parallel profiles "Sketch40" along 1 edges at (457.2, 106.426, -9.144) section 1 on bodies 3 bodies 3 in component "Back"
ref_plane "WorkPlane36" through (457.2, 11.938, -18.288) normal (0, 0, 1) x (1, 0, 0)
sketch "Sketch41" plane through (457.2, 11.938, -18.288) normal (0, 0, 1) x (1, 0, 0)
  line L0 (0, 0) -> (147.9099, 0) construction
  line L1 (0, -13.7979) -> (0, 0) construction
  line L2 (0, 0) -> (2.2451, -2.2451) construction
  circle A0 centre (2.2451, -2.2451) radius 3.175
  dimension "d350" = 3.175
  constraint coincident L0.start L1.end
  constraint coincident L0.start A0
  measures "d350" distance of L0.start L2.end
sweep "Sweep16'" cut kept parallel profiles "Sketch41" along 1 edges at (457.2, 11.938, -9.144) section 1 on bodies 3 bodies 3 in component "Back"
component "Shelf" placed x (1, 0, 0) y (0, 1, 0) z (0, 0, 1) at (0, 0, 0)
component "Side" placed x (1, 0, 0) y (0, 1, 0) z (0, 0, 1) at (0, 0, 0)
component "Shelf" placed x (1, 0, 0) y (0, 1, 0) z (0, 0, 1) at (0, 94.488, 0)
component "Shelf" placed x (1, 0, 0) y (0, 1, 0) z (0, 0, 1) at (0, 188.976, 0)
component "Shelf" placed x (1, 0, 0) y (0, 1, 0) z (0, 0, 1) at (0, 283.464, 0)
component "Side" placed x (1, 0, 0) y (0, 1, 0) z (0, 0, 1) at (-1085.088, 0, 0)
component "Back" placed x (1, 0, 0) y (0, 1, 0) z (0, 0, 1) at (0, 0, 0)
equation "d8 = ( 3.25 / 2 ) * 1 in"
equation "pigmentdiam = 2.85 in"
equation "d10 = pigmentdiam"
equation "distance = 0"
equation "d20 = 0.25 in / 2 + 0.00 in"
equation "DistanceOne = 1"
equation "d28 = 0.25 in / 2 + 0.00 in"
equation "d42 = 4.72 in + 0.25 in"
equation "d67 = 0.25 in / 2 + 0.00 in"
equation "d75 = 0.25 in / 2 + 0.00 in"
equation "d83 = 0.25 in / 2 + 0.00 in"
equation "d91 = 0.25 in / 2 + 0.00 in"
equation "d99 = 0.25 in / 2 + 0.00 in"
equation "d107 = 0.25 in / 2 + 0.00 in"
equation "d115 = 0.25 in / 2 + 0.00 in"
equation "d123 = 0.25 in / 2 + 0.00 in"
equation "d131 = 0.25 in / 2 + 0.00 in"
equation "d139 = 0.25 in / 2 + 0.00 in"
equation "d147 = 0.25 in / 2 + 0.00 in"
equation "d155 = 0.25 in / 2 + 0.00 in"
equation "d163 = 0.25 in / 2 + 0.00 in"
equation "d171 = 0.25 in / 2 + 0.00 in"
equation "d179 = 0.25 in / 2 + 0.00 in"
equation "d187 = 0.25 in / 2 + 0.00 in"
equation "d195 = 0.25 in / 2 + 0.00 in"
equation "d203 = 0.25 in / 2 + 0.00 in"
equation "d230 = 0.25 in / 2 + 0.00 in"
equation "d238 = 0.25 in / 2 + 0.00 in"
equation "d246 = 0.25 in / 2 + 0.00 in"
equation "d254 = 0.25 in / 2 + 0.00 in"
equation "d262 = 0.25 in / 2 + 0.00 in"
equation "d270 = 0.25 in / 2 + 0.00 in"
equation "d278 = 0.25 in / 2 + 0.00 in"
equation "d286 = 0.25 in / 2 + 0.00 in"
equation "d294 = 0.25 in / 2 + 0.00 in"
equation "d302 = 0.25 in / 2 + 0.00 in"
equation "d310 = 0.25 in / 2 + 0.00 in"
equation "d318 = 0.25 in / 2 + 0.00 in"
equation "d326 = 0.25 in / 2 + 0.00 in"
equation "d334 = 0.25 in / 2 + 0.00 in"
equation "d342 = 0.25 in / 2 + 0.00 in"
equation "d350 = 0.25 in / 2 + 0.00 in"
